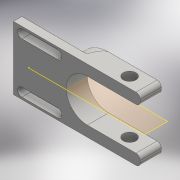
# Autodesk Inventor part: Y-pulley-mount
Saved by Autodesk Inventor 2016 (Build 200138000, 138)
## iProperties
Created: 2015-05-19
Part Number: Y-pulley-mount
Material: Generic
Document SubType Name: Modeling
Designer: as
Mass: 6.35429 g
Surface Area: 44.4083 cm^2
Volume: 6.35429 cm^3
Density: 1 g/cm^3
Appearance: Default
Author: as
Autodesk Inventor part; units mm, degrees
ref_plane "YZ Plane" through (0, 0, 0) normal (1, 0, 0) x (0, 1, 0)
ref_plane "XZ Plane" through (0, 0, 0) normal (0, 1, 0) x (-1, 0, 0)
ref_plane "XY Plane" through (0, 0, 0) normal (0, 0, 1) x (1, 0, 0)
sketch "Sketch1" plane through (0, 0, 0) normal (0, 0, 1) x (1, 0, 0)
  line L0 (0, 0) -> (-60, 0)
  line L1 (-60, 0) -> (-60, -10)
  line L2 (-60, -10) -> (0, -10)
  line L3 (0, -10) -> (0, 0)
  circle A0 centre (-10, -5) radius 3
  dimension "d0" = 60
  dimension "d1" = 6
  constraints: 8 end point, 2 parallel, 1 centre point, 1 horizontal, 1 perpendicular
  measures "d0" distance of L2.end L1.end
  measures "d1" diameter of A0
extrude "Extrusion1" add sketch "Sketch1" along normal blind 30
sketch "Sketch2" plane through (-60, -10, 0) normal (0, -1, 0) x (1, 0, 0)
  line L0 (60, 0) -> (60, 30) projected
  line L1 (60, 15) -> (35, 15) construction
  line L2 (60, 25) -> (35, 25)
  line L3 (35, 5) -> (60, 5)
  arc A0 (60, 5) -> (60, 25) centre (60, 15) ccw
  arc A1 (35, 25) -> (35, 5) centre (35, 15) ccw
  line L4 (0, 0) -> (60, 0) projected
  point P0 (47.5, 15)
  dimension "d4" = 25
  dimension "d5" = 20
  dimension "d6" = 15
  constraints: 8 end point, 4 point on circle, 4 tangent, 2 centre point, 2 midpoint, 1 horizontal, 1 parallel
  measures "d4" distance of L1.start L1.end
  measures "d5" diameter of A1
  measures "d6" distance between parallel lines of L4 L1
extrude "Extrusion2" cut sketch "Sketch2" against normal through all
sketch "Sketch3" plane through (-60, 0, 0) normal (0, 1, 0) x (1, 0, 0)
  line L0 (2, -3.05) -> (23, -3.05) construction
  line L1 (4.05, -5.1) -> (20.95, -5.1)
  line L2 (20.95, -1) -> (4.05, -1)
  arc A0 (4.05, -1) -> (4.05, -5.1) centre (4.05, -3.05) ccw
  arc A1 (20.95, -5.1) -> (20.95, -1) centre (20.95, -3.05) ccw
  line L3 (0, 0) -> (60, 0) projected
  line L4 (0, 0) -> (0, -30) projected
  point P0 (12.5, -3.05)
  dimension "d9" = 4.1
  dimension "d10" = 1
  dimension "d14" = 2
  dimension "d15" = 23
  constraints: 8 end point, 6 point on circle, 4 tangent, 2 centre point, 2 point on line, 1 horizontal, 1 midpoint, 1 parallel
  measures "d9" diameter of A1
  measures "d10" distance between parallel lines of L3 L2
  measures "d14" distance from line of L4 L0.start
  measures "d15" distance from line of L4 L0.end
extrude "Extrusion3" cut sketch "Sketch3" against normal through all
ref_plane "Work Plane1" through (0, 0, 15) normal (0, 0, 1) x (1, 0, 0)
mirror "Mirror1" about plane through (0, 0, 15) normal (0, 0, 1) of "Extrusion3"
sketch "Sketch4" plane through (-60, 0, 0) normal (0, 1, 0) x (1, 0, 0)
  arc A0 (35, -5) -> (35, -25) centre (35, -15) ccw projected
  arc A1 (35, 0) -> (35, -30) centre (35, -15) ccw
  line L0 (0, 0) -> (0, -30) projected
  line L1 (35, -30) -> (0, -30)
  line L2 (0, -30) -> (0, 0)
  line L3 (0, 0) -> (35, 0)
  point P0 (60, 0)
  constraints: 6 end point, 2 perpendicular, 2 point on circle, 1 centre point, 1 horizontal
extrude "Extrusion4" cut sketch "Sketch4" against normal blind 6
chamfer "Chamfer1" distance 6 angle 6 1 edges at (-40, -6, 15) measured on face at (-40, -5.5, 15)
fillet "Fillet1" radius 2 4 edges at (0, -5, 0) (0, -5, 5) (0, -5, 25) (0, -5, 30)
sketch "Sketch5" plane through (-60, -10, 0) normal (-1, 0, 0) x (0, 0, 1)
  line L0 (30, 4) -> (0, 4) projected
  line L1 (0, 0) -> (30, 0)
  line L2 (30, 0) -> (30, 4)
  line L3 (30, 4) -> (0, 4)
  line L4 (0, 4) -> (0, 0)
  point P0 (0, 10)
  constraints: 8 end point, 2 parallel, 1 horizontal, 1 perpendicular
sketch "Sketch6" plane through (-60, -6, 0) normal (0, 1, 0) x (1, 0, 0)
  line L0 (-5, 0) -> (30.605, 0) projected
  line L1 (-5, 0) -> (-5, -30) projected
  line L2 (0, 0) -> (-5, 0)
  line L3 (-5, 0) -> (-5, -30)
  line L4 (-5, -30) -> (0, -30)
  line L5 (0, -30) -> (0, 0)
  point P0 (60, 0)
  constraints: 8 end point, 2 parallel, 1 horizontal, 1 perpendicular, 1 point on line
sketch "Sketch7" plane through (-60, -6, 30) normal (1, 0, 0) x (0, 0, -1)
  line L0 (0, -4) -> (0, 6) projected
  line L1 (30, -4) -> (30, 6) projected
  line L2 (0, 0) -> (30, 0)
  line L3 (30, 0) -> (30, 6)
  line L4 (30, 6) -> (0, 6)
  line L5 (0, 6) -> (0, 0)
  constraints: 8 end point, 2 parallel, 1 horizontal, 1 perpendicular, 1 point on line
equation "\"d6\" = 0.5 * d2"
equation "\"d13\" = -0.5 * d2"
equation "\"d2\" = 30"
body "Solid1"
